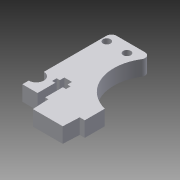
# Autodesk Inventor part: yCarWireHolder
Saved by Autodesk Inventor 2013 (Build 170138000, 138)
## iProperties
Created: 2015-01-14
Part Number: yCarWireHolder
Material: Generic
Document SubType Name: Modeling
Designer: dzban
Density: 1 g/cm^3
Author: dzban
Autodesk Inventor part; units mm, degrees
ref_plane "YZ Plane" through (0, 0, 0) normal (1, 0, 0) x (0, 1, 0)
ref_plane "XZ Plane" through (0, 0, 0) normal (0, 1, 0) x (-1, 0, 0)
ref_plane "XY Plane" through (0, 0, 0) normal (0, 0, 1) x (1, 0, 0)
sketch "Sketch1" plane through (0, 0, 0) normal (0, 0, 1) x (1, 0, 0)
  arc A0 (-22.65, 35.1889) -> (-24.65, 33.1889) centre (-22.65, 33.1889) ccw
  line L0 (-24.65, 8.5016) -> (-24.65, 33.1889)
  arc A1 (-24.65, 2.5016) -> (-24.65, 8.5016) centre (-24.65, 5.5016) ccw
  line L1 (-24.65, 0) -> (-24.65, 2.5016)
  line L2 (-18.65, 0) -> (-24.65, 0)
  line L3 (-18.65, 7) -> (-18.65, 0)
  line L4 (-19.9, 7) -> (-18.65, 7)
  line L5 (-19.9, 8.8) -> (-19.9, 7)
  line L6 (-18.65, 8.8) -> (-19.9, 8.8)
  line L7 (-18.65, 10.6) -> (-18.65, 8.8)
  line L8 (-15.65, 10.6) -> (-18.65, 10.6)
  line L9 (-15.65, 8.8) -> (-15.65, 10.6)
  line L10 (-14.4, 8.8) -> (-15.65, 8.8)
  line L11 (-14.4, 7) -> (-14.4, 8.8)
  line L12 (-15.65, 7) -> (-14.4, 7)
  line L13 (-15.65, 0) -> (-15.65, 7)
  line L14 (-14.4, 0) -> (-15.65, 0)
  line L15 (-14.1, -6.4) -> (-14.4, 0)
  line L16 (-2.3, -6.4) -> (-14.1, -6.4)
  line L17 (-2, 0) -> (-2.3, -6.4)
  line L18 (0, 0) -> (-2, 0)
  line L19 (0, 7.9) -> (0, 0)
  arc A2 (-9.6633, 32.1341) -> (0, 7.9) centre (4.112, 23.5833) ccw
  arc A3 (-9.6633, 32.1341) -> (-11.3625, 35.1889) centre (-11.3625, 33.1889) ccw
  line L20 (-22.65, 35.1889) -> (-11.3625, 35.1889)
  circle A4 centre (-14.65, 31.341) radius 1.5
  circle A5 centre (-22.65, 31.341) radius 1.5
  constraints: 42 end point, 8 point on circle, 6 centre point
extrude "Extrusion1" add sketch "Sketch1" along normal blind 6
body "Solid1"
